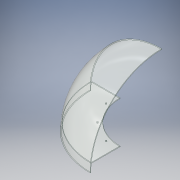
# Autodesk Inventor part: shell
Saved by Autodesk Inventor 2019 (Build 230136000, 136)
## iProperties
Created: 2019-02-10
Part Number: shell
Material: Glass
Document SubType Name: Modeling
Designer: mashimaro
Density: 2.18 g/cm^3
Appearance: Clear
Author: mashimaro
Autodesk Inventor part; units mm, degrees
ref_plane "YZ Plane" through (0, 0, 0) normal (1, 0, 0) x (0, 1, 0)
ref_plane "XZ Plane" through (0, 0, 0) normal (0, 1, 0) x (-1, 0, 0)
ref_plane "XY Plane" through (0, 0, 0) normal (0, 0, 1) x (1, 0, 0)
sketch "Sketch1" plane through (0, 0, 0) normal (0, 1, 0) x (-1, 0, 0)
  arc A0 (172, 0) -> (0, 172) centre (0, 0) ccw
  line L0 (0, 172) -> (0, 0)
  line L1 (172, 0) -> (0, 0)
  constraints: 4 end point, 2 point on circle, 1 centre point, 1 horizontal, 1 vertical
revolve "Revolution1" add sketch "Sketch1" angle 90 about axis through (0, 0, 172) along (0, 0, -1)
sketch "Sketch2" plane through (-172, 0, 0) normal (0, -1, 0) x (1, 0, 0)
  arc A0 (172, 170) -> (2, 0) centre (172, 0) ccw
  line L0 (172, 0) -> (172, 172) projected
  line L1 (172, 0) -> (2, 0)
  line L2 (172, 0) -> (172, 170)
  constraints: 4 end point, 2 point on circle, 1 centre point, 1 coincident, 1 perpendicular, 1 point on line
revolve "Revolution2" cut sketch "Sketch2" angle 90 about axis through (0, 0, 0) along (0, 0, -1)
sketch "Sketch3" plane through (0, 0, 0) normal (1, 0, 0) x (0, -0.7071068, -0.7071068)
  arc A0 (-121.6224, 121.6224) -> (-121.6224, -121.6224) centre (0, 0) ccw projected
  arc A1 (-120.2082, 120.2082) -> (-120.2082, -120.2082) centre (0, 0) ccw projected
  line L0 (-121.6224, -121.6224) -> (-101.6224, -121.6224) construction
  line L1 (0, 0) -> (-121.6224, 121.6224) projected
  line L2 (0, 0) -> (-14.1421, 14.1421)
  line L3 (-84.8528, -56.5685) -> (-133.5155, -105.2312)
  line L4 (-84.8528, -56.5685) -> (-83.4386, -57.9828)
  line L5 (-83.4386, -57.9828) -> (-132.2603, -106.8045)
  point P0 (-134.7537, -103.641)
  dimension "d49" = 2
  constraints: 10 end point, 3 point on circle, 1 horizontal, 1 perpendicular, 1 point on line
  measures "d49" distance of L3.start L4.end
revolve "Revolution3" add sketch "Sketch3" angle 90 about axis through (0, 0, 0) along (0, -1, 0)
sketch "Sketch7" plane through (0, 20, 168.8194) normal (0, 1, 0) x (1, 0, 0)
  circle A0 centre (-27.763, 63.2747) radius 1.5
  circle A1 centre (-77.0746, 91.7448) radius 1.5
  circle A2 centre (-105.5447, 141.0564) radius 1.5
  line L0 (-77.7817, 91.0377) -> (-77.0746, 91.7448)
  line L1 (-77.7817, 91.0377) -> (-76.7817, 91.0377) construction
  dimension "d57" = 3
  dimension "d58" = 3
  dimension "d59" = 3
  dimension "d62" = 1
  dimension "d63" = 45
  constraints: 4 end point, 3 centre point, 1 equal length, 1 horizontal
  measures "d57" diameter of A0
  measures "d58" diameter of A1
  measures "d59" diameter of A2
  measures "d62" distance of L0.start L0.end
  measures "d63" angle of L1 L0
extrude "Extrusion4" cut sketch "Sketch7" against normal blind 10
body "Solid1"
